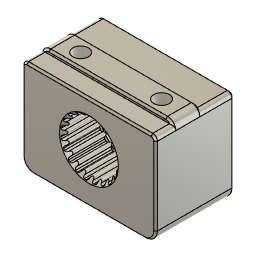
nozzle_probe (Autodesk Fusion 360 design; units mm, degrees)
Autodesk Fusion 360 part; units mm, degrees
sketch "Sketch1" plane through (0, 0, 0) normal (0, 0, 1) x (1, 0, 0)
  line L0 (14.5, -10.2) -> (-14.5, -10.2)
  line L1 (-14.5, -10.2) -> (-14.5, 10.2)
  line L2 (-14.5, 10.2) -> (14.5, 10.2)
  line L3 (14.5, 10.2) -> (14.5, -10.2)
  line L4 (14.5, -10.2) -> (-14.5, 10.2) construction
  line L5 (-14.5, -10.2) -> (14.5, 10.2) construction
  circle A0 centre (0, 0.6) radius 6.26
  dimension "d115" = 29
  dimension "d116" = 20.4
  dimension "d117" = 12.52
  dimension "d177" = 10.8
  constraint horizontal L0
  constraint perpendicular L0 L1
  constraint parallel L0 L2
  constraint parallel L1 L3
  constraint coincident L4 origin
  constraint coincident L5 origin
  constraint vertical origin A0.centre
  measures "d115" distance of L1.end L2.end
  measures "d116" distance of L0.start L2.end
  measures "d117" diameter of A0
  measures "d177" distance of L0 A0.centre
extrude "Extrude1" add sketch "Sketch1" along normal blind 17 contours L0 L1 L2 L3 | A0
sketch "Sketch6" plane through (0, 0, 17) normal (0, 0, 1) x (1, 0, 0)
  line L0 (14.5, 10.2) -> (-14.5, 10.2)
  line L1 (-14.5, 10.2) -> (-14.5, -10.2)
  line L2 (-14.5, -10.2) -> (14.5, -10.2)
  line L3 (14.5, -10.2) -> (14.5, 10.2)
  circle A0 centre (0, 0.6) radius 6.26
extrude "Extrude6" cut sketch "Sketch6" against normal blind 8 contours A0
sketch "Sketch7" plane through (0, 0, 17) normal (0, 0, 1) x (1, 0, 0)
  circle A0 centre (0, 0.6) radius 6.26
  line L0 (14.5, 10.2) -> (-14.5, 10.2)
  line L1 (-14.5, 10.2) -> (-14.5, -10.2)
  line L2 (-14.5, -10.2) -> (14.5, -10.2)
  line L3 (14.5, -10.2) -> (14.5, 10.2)
  circle A1 centre (0, 0.6) radius 6.26
  circle A2 centre (0, 0.6) radius 5.2
  dimension "d179" = 10.4
  constraint coincident A0.centre A1.centre
  measures "d179" diameter of A2
extrude "Extrude8" cut sketch "Sketch7" against normal blind 9 contours A2
sketch "Sketch2" plane through (0, 0, 17) normal (0, 0, 1) x (1, 0, 0)
  line L0 (14.5, 10.2) -> (-14.5, 10.2)
  line L1 (-14.5, 10.2) -> (-14.5, -10.2)
  line L2 (-14.5, -10.2) -> (14.5, -10.2)
  line L3 (14.5, -10.2) -> (14.5, 10.2)
  line L4 (0.4, 6.47) -> (0.4, 6.8472)
  line L5 (-0.4, 6.8472) -> (-0.4, 6.47)
  arc A0 (-0.4, 6.47) -> (0.4, 6.47) centre (0, 6.47) ccw
  circle A1 centre (0, 0.6) radius 6.26
  circle A2 centre (0, 0.6) radius 6.26
  dimension "d121" = 0.8
  dimension "d172" = 5.87
  constraint vertical L4
  constraint vertical L5
  constraint tangent L4 A0
  constraint tangent L5 A0
  constraint vertical A0.centre A1.centre
  constraint coincident L4.end A2
  constraint coincident L5.start A2
  measures "d121" diameter of A0
  measures "d172" distance of A0.centre A1.centre
extrude "Extrude2" add sketch "Sketch2" against normal blind 8 contours L4 L5 A0 A1 A2 picked at (-0.0445, 6.5995)
fillet "Fillet1" radius 0.35 2 edges at (-0.4, 6.8472, 13) (0.4, 6.8472, 13)
chamfer "Chamfer1" distance 0.4 angle 45 1 edges at (-4.8481, 2.4804, 9)
pattern_circular "C-Pattern1" count 20 over 360 about axis through (0, 0.6, 17) along (0, 0, -1) of 3 faces at (-0.5335, 6.7373, 14.3333) (-0.0042, 6.07, 14.2901) (0.5475, 6.7477, 14.3333)
sketch "Sketch3" plane through (0, 0, 0) normal (1, 0, 0) x (0, 0, -1)
  line L0 (-17, 7) -> (-15, 5)
  line L1 (-15, 5) -> (-17, 5)
  line L2 (-17, 5) -> (-17, 7)
  line L3 (-17, -10.2, -14.5) -> (-17, -10.2, 14.5)
  line L4 (-17, 10.2) -> (-17, 0.6)
  line L5 (-17, 0.6) -> (-17, 7)
  line L6 (-17, 6.3024) -> (-17, 5.7827)
  line L7 (-17, 6.751) -> (-17, 6.3024)
  line L8 (-17, 6.751) -> (-17, 6.8094)
  line L9 (-17, 6.8122) -> (-17, 6.4659)
  line L10 (-17, 6.4659) -> (-17, 6.8122)
  line L11 (-17, 6.751) -> (-17, 6.8094)
  line L12 (-17, 6.2936) -> (-17, 6.0552)
  line L13 (-17, 6.751) -> (-17, 6.3024)
  line L14 (-17, 6.0904) -> (-17, 5.5807)
  line L15 (-17, 5.5807) -> (-17, 4.9489)
  line L16 (-17, 5.2518) -> (-17, 5.1105)
  line L17 (-17, 4.8925) -> (-17, 5.1566)
  line L18 (-17, 4.8925) -> (-17, 4.3715)
  line L19 (-17, 4.3715) -> (-17, 3.6503)
  line L20 (-17, 3.789) -> (-17, 3.6071)
  line L21 (-17, 3.2743) -> (-17, 3.6071)
  line L22 (-17, 3.2743) -> (-17, 2.7931)
  line L23 (-17, 2.7931) -> (-17, 2.0139)
  line L24 (-17, 2.0483) -> (-17, 1.7633)
  line L25 (-17, 1.3944) -> (-17, 1.7633)
  line L26 (-17, 0.2) -> (-17, -0.1944)
  line L27 (-17, 1) -> (-17, 0.2)
  line L28 (-17, 1.3944) -> (-17, 1)
  line L29 (-17, -0.5633) -> (-17, -0.8483)
  line L30 (-17, -0.8139) -> (-17, -1.5931)
  line L31 (-17, -1.5931) -> (-17, -2.0743)
  line L32 (-17, -2.4071) -> (-17, -2.0743)
  line L33 (-17, -2.4071) -> (-17, -2.589)
  line L34 (-17, -2.4503) -> (-17, -3.1715)
  line L35 (-17, -3.1715) -> (-17, -3.6925)
  line L36 (-17, -3.9566) -> (-17, -3.6925)
  line L37 (-17, -3.9105) -> (-17, -4.0518)
  line L38 (-17, -3.7489) -> (-17, -4.3807)
  line L39 (-17, -4.3807) -> (-17, -4.8904)
  line L40 (-17, -5.06) -> (-17, -4.8904)
  line L41 (-17, -4.8552) -> (-17, -5.0936)
  line L42 (-17, -4.5827) -> (-17, -5.1024)
  line L43 (-17, -5.1024) -> (-17, -5.551)
  line L44 (-17, -5.6094) -> (-17, -5.551)
  line L45 (-17, -5.2659) -> (-17, -5.6122)
  line L46 (-17, -4.87) -> (-17, -5.2659)
  line L47 (-17, -5.2659) -> (-17, -5.6122)
  line L48 (-17, -5.6094) -> (-17, -5.551)
  line L49 (-17, -5.1024) -> (-17, -5.551)
  line L50 (-17, -4.5827) -> (-17, -5.1024)
  line L51 (-17, -4.8552) -> (-17, -5.0936)
  line L52 (-17, -5.06) -> (-17, -4.8904)
  line L53 (-17, -4.3807) -> (-17, -4.8904)
  line L54 (-17, -3.7489) -> (-17, -4.3807)
  line L55 (-17, -3.9105) -> (-17, -4.0518)
  line L56 (-17, -3.9566) -> (-17, -3.6925)
  line L57 (-17, -3.1715) -> (-17, -3.6925)
  line L58 (-17, -2.4503) -> (-17, -3.1715)
  line L59 (-17, -2.4071) -> (-17, -2.589)
  line L60 (-17, -2.4071) -> (-17, -2.0743)
  line L61 (-17, -1.5931) -> (-17, -2.0743)
  line L62 (-17, -0.8139) -> (-17, -1.5931)
  line L63 (-17, -0.5633) -> (-17, -0.8483)
  line L64 (-17, -0.5633) -> (-17, -0.1944)
  line L65 (-17, 1.3944) -> (-17, 1)
  line L66 (-17, 1) -> (-17, 0.2)
  line L67 (-17, 0.2) -> (-17, -0.1944)
  line L68 (-17, 2.0483) -> (-17, 1.7633)
  line L69 (-17, 2.7931) -> (-17, 2.0139)
  line L70 (-17, 3.2743) -> (-17, 2.7931)
  line L71 (-17, 3.2743) -> (-17, 3.6071)
  line L72 (-17, 3.789) -> (-17, 3.6071)
  line L73 (-17, 4.3715) -> (-17, 3.6503)
  line L74 (-17, 4.8925) -> (-17, 4.3715)
  line L75 (-17, 4.8925) -> (-17, 5.1566)
  line L76 (-17, 5.2518) -> (-17, 5.1105)
  line L77 (-17, 5.5807) -> (-17, 4.9489)
  line L78 (-17, 6.0904) -> (-17, 5.5807)
  line L79 (-17, 6.0904) -> (-17, 6.26)
  line L80 (-17, 6.2936) -> (-17, 6.0552)
  line L81 (-17, 6.0904) -> (-17, 6.26)
  line L82 (-17, -0.5633) -> (-17, -0.1944)
  line L83 (-17, 1.3944) -> (-17, 1.7633)
  point P0 (-17, 10.2)
  point P1 (-17, -10.2)
  dimension "d129" = 2
  dimension "d163" = 9.6
  dimension "d164" = 6.4
  constraint perpendicular L1 L2
  constraint equal L1 L2
  constraint vertical L2
  constraint coincident P0 L4.start
  constraint vertical L4
  constraint vertical L5
  constraint coincident L2 L0.start
  constraint coincident L0.start L2.end
  measures "d129" distance of L0.start L1.end
  measures "d163" distance of P0 L4.end
  measures "d164" distance of L4.end L0.start
revolve "Revolve1" cut sketch "Sketch3" angle 360 about axis through (0, 0.6, 17) along (0, 0, 1)
hole "Hole1" at (-8.8, -10.2, 10) direction (0, 1, 0) diameter 3.4 end through all counterbore diameter 6 counterbore depth 5
pattern_linear "R-Pattern1" count 2 spacing 17.6 along (1, 0, 0) of "Hole1"
sketch "Sketch4" plane through (0, -10.2, 0) normal (0, -1, 0) x (1, 0, 0)
  circle A0 centre (-8.8, 10) radius 3
  line L0 (14.5, 17) -> (-14.5, 17)
  line L1 (-14.5, 17) -> (-14.5, 0)
  line L2 (-14.5, 0) -> (14.5, 0)
  line L3 (14.5, 0) -> (14.5, 17)
  line L4 (-2.3342, 4.8) -> (1.0842, 10)
  line L5 (1.0842, 10) -> (2.3342, 10)
  line L6 (2.3342, 10) -> (-1.0842, 4.8)
  line L7 (-1.0842, 4.8) -> (-2.3342, 4.8)
  line L8 (0.0342, 10) -> (-1.2158, 10)
  line L9 (-1.2158, 10) -> (-2.925, 7.4)
  line L10 (-2.925, 7.4) -> (-1.675, 7.4)
  line L11 (-1.675, 7.4) -> (0.0342, 10)
  line L12 (1.675, 7.4) -> (2.925, 7.4)
  line L13 (-0.0342, 4.8) -> (1.675, 7.4)
  line L14 (2.925, 7.4) -> (1.2158, 4.8)
  line L15 (1.2158, 4.8) -> (-0.0342, 4.8)
  line L16 (1.0842, 10) -> (-1.0842, 4.8) construction
  line L17 (-2.3342, 4.8) -> (2.3342, 10) construction
  circle A1 centre (8.8, 10) radius 3
  point P0 (0, 7.4)
  dimension "d146" = 5.2
  dimension "d147" = 1.25
  dimension "d148" = 1.05
  dimension "d149" = 2.6
  dimension "d150" = 1.05
  dimension "d151" = 7.4
  dimension "d152" = 14.5
  dimension "d209" = 56.68
  constraint horizontal L5
  constraint horizontal L7
  constraint parallel L4 L6
  constraint parallel L5 L8
  constraint parallel L4 L9
  constraint parallel L5 L10
  constraint parallel L4 L11
  constraint equal L5 L8
  constraint horizontal L12
  constraint parallel L6 L13
  constraint parallel L13 L14
  constraint horizontal L15
  constraint collinear L7 L15
  constraint collinear L10 L12
  constraint equal L10 L15
  constraint midpoint L17 P0
  constraint collinear L5 L8
  measures "d146" distance of L5 L7
  measures "d147" distance of L4.end L5.end
  measures "d148" horizontal distance of L4.end L8.start
  measures "d149" distance of L8 L10
  measures "d150" distance of L6.end L13.start
  measures "d151" distance of L2 P0
  measures "d152" distance of L1 P0
  measures "d209" angle of L4 L7
extrude "Extrude3" cut sketch "Sketch4" against normal blind 1.6 contours L4 L5 L6 L7 | L8 L9 L10 L11 | L12 L13 L14 L15
sketch "Sketch5" plane through (0, 0, 0) normal (0, 0, -1) x (-1, 0, 0)
  line L0 (3.1, -7.8) -> (-3.1, -7.8)
  line L1 (-3.1, -7.8) -> (-3.1, 5.4)
  line L2 (3.1, 5.4) -> (3.1, -7.8)
  line L3 (14.5, -6.4) -> (3.1, -6.4)
  line L4 (3.1, -6.4) -> (3.1, 4)
  line L5 (3.1, 4) -> (14.5, 4)
  line L6 (14.5, 4) -> (14.5, -6.4)
  line L7 (-3.1, 5.4) -> (3.1, 5.4)
  line L8 (14.5, 10.2) -> (-14.5, 10.2)
  line L9 (-14.5, 10.2) -> (-14.5, -10.2)
  line L10 (-14.5, -10.2) -> (14.5, -10.2)
  line L11 (14.5, -10.2) -> (14.5, 10.2)
  line L12 (-3.1, -4.5) -> (3.1, -4.5)
  dimension "d156" = 6.2
  dimension "d157" = 13.2
  dimension "d158" = 11.4
  dimension "d159" = 10.4
  dimension "d160" = 1.4
  dimension "d175" = 9.9
  constraint horizontal L3
  constraint horizontal L5
  constraint vertical L6
  constraint coincident L2 L4.end
  constraint vertical L2
  constraint vertical L4
  constraint vertical L1
  constraint horizontal L7
  constraint coincident L1 L12.start
  constraint coincident L4 L12.end
  constraint horizontal L12
  measures "d156" distance of L0.start L0.end
  measures "d157" distance of L0.end L1.end
  measures "d158" distance of L3.start L3.end
  measures "d159" distance of L3.start L5.end
  measures "d160" distance of L0 L3
  measures "d175" distance of L7 L12
extrude "Extrude4" cut sketch "Sketch5" against normal blind 8.2 contours L0 L1 L2 L4 L12 | L1 L2 L4 L7 L12
extrude "Extrude5" cut sketch "Sketch5" against normal blind 6 contours L2 L3 L4 L5 L6 L11
extrude "Extrude7" cut sketch "Sketch5" against normal blind 9 contours L1 L2 L4 L7 L12
sketch "Sketch8" plane through (-14.5, -0.131, 0.0085) normal (-1, 0, 0) x (0, 0, 1)
  line L0 (-0.0085, 4.131) -> (5.9915, 4.131)
  line L1 (5.9915, 4.131) -> (5.9915, -6.269)
  line L2 (5.9915, -6.269) -> (-0.0085, -6.269)
  line L3 (-0.0085, -6.269) -> (-0.0085, -10.069)
  line L4 (-0.0085, -10.069) -> (16.9915, -10.069)
  line L5 (16.9915, -10.069) -> (16.9915, 10.331)
  line L6 (16.9915, 10.331) -> (-0.0085, 10.331)
  line L7 (-0.0085, 10.331) -> (-0.0085, 4.131)
  line L8 (5.9915, 4.131) -> (5.9915, -6.269)
  line L9 (5.9915, -1.069) -> (12.5209, -1.069)
  line L10 (5.9915, -2.844) -> (8.7915, -2.844)
  line L11 (8.7915, -2.844) -> (8.7915, 0.706)
  line L12 (8.7915, 0.706) -> (5.9915, 0.706)
  line L13 (5.9915, 0.706) -> (5.9915, -2.844)
  line L14 (5.9915, -2.844) -> (8.7915, 0.706) construction
  line L15 (8.7915, -2.844) -> (5.9915, 0.706) construction
  point P0 (7.3915, -1.069)
  dimension "d183" = 3.55
  dimension "d184" = 2.8
  constraint midpoint L1 L9.start
  constraint perpendicular L1 L9
  constraint horizontal L10
  constraint perpendicular L10 L11
  constraint parallel L10 L12
  constraint parallel L11 L13
  constraint coincident L14 P0
  constraint coincident L15 P0
  constraint coincident L9 P0
  constraint coincident L1 L10.start
  measures "d183" distance of L10.end L11.end
  measures "d184" distance of L10.start L10.end
extrude "Extrude9" cut sketch "Sketch8" against normal blind 3.4 contours L1 L8 L9 L11 L12 L13 | L1 L8 L9 L10 L11 L13
fillet "Fillet2" radius 1 2 edges at (-12.8, 0.575, 8.8) (-12.8, -2.975, 8.8)
hole "Hole2" at (3.1, 2.05, 3) direction (1, 0, 0) diameter 1.6 depth 5.6 tip angle 180
pattern_linear "R-Pattern2" count 2 spacing 6.5 along (0, -1, 0) of "Hole2"
sketch "Sketch9" plane through (0, 10.2, 0) normal (0, 1, 0) x (-1, 0, 0)
  circle A0 centre (-8.8, 10) radius 1.7
  circle A1 centre (8.8, 10) radius 1.7
  line L0 (-14.5, 0) -> (14.5, 0)
  line L1 (14.5, 0) -> (14.5, 17)
  line L2 (14.5, 17) -> (-14.5, 17)
  line L3 (-14.5, 17) -> (-14.5, 0)
  line L4 (-14.5, 13) -> (14.5, 13)
  line L5 (14.5, 13) -> (14.5, 7)
  line L6 (14.5, 7) -> (-14.5, 7)
  line L7 (-14.5, 7) -> (-14.5, 13)
  dimension "d198" = 7
  dimension "d199" = 6
  constraint horizontal L4
  constraint vertical L5
  constraint horizontal L6
  constraint vertical L7
  constraint coincident L1 L5.end
  constraint coincident L3 L4.start
  measures "d198" distance of L0 L6
  measures "d199" distance of L4.end L5.end
extrude "Extrude10" add sketch "Sketch9" along normal blind 0.8 contours L1 L3 L4 L5 L6 L7
fillet "Fillet3" radius 2.5 2 edges at (-14.5, -10.2, 8.5) (14.5, -10.2, 8.5)
fillet "Fillet3" radius 1 4 edges at (14.5, 10.2, 15) (14.5, 10.2, 3.5) (-14.5, 10.2, 15) (-14.5, 10.2, 3.5)
fillet "Fillet3" radius 1.8 2 edges at (-14.5, 11, 10) (14.5, 11, 10)
chamfer "Chamfer2" distance 0.4 angle 45 30 edges at (0, 11, 13) (-13.9728, 10.4728, 13) (13.9728, 10.4728, 13) (0, 11, 7) (13.9728, 10.4728, 7) (-13.9728, 10.4728, 7) (0, 10.2, 17) (-14.2071, 9.9071, 17) (-14.5, 0.75, 17) (-13.7678, -9.4678, 17) (0, -10.2, 17) (13.7678, -9.4678, 17) (14.5, 0.75, 17) (14.2071, 9.9071, 17) (0, 10.2, 0) (14.2071, 9.9071, 0) (14.5, 0.75, 0) (13.7678, -9.4678, 0) (0, -10.2, 0) (-13.7678, -9.4678, 0) (-14.5, -7.05, 0) (-14.5, 6.6, 0) (-14.2071, 9.9071, 0) (-3.1, 4.7, 0) (-8.8, 4, 0) (0, 5.4, 0) (3.1, -1.2, 0) (0, -7.8, 0) (-3.1, -7.1, 0) (-8.8, -6.4, 0)
sketch "Sketch10" plane through (0, 0, 6) normal (0, 0, -1) x (-1, 0, 0)
  line L0 (14.5, -2.975) -> (11.1, -2.975)
  line L1 (11.1, -2.975) -> (11.1, 0.575)
  line L2 (11.1, 0.575) -> (14.5, 0.575)
  line L3 (14.5, 0.575) -> (14.5, 4)
  line L4 (14.5, 4) -> (3.1, 4)
  line L5 (3.1, 4) -> (3.1, -6.4)
  line L6 (3.1, -6.4) -> (14.5, -6.4)
  line L7 (14.5, -6.4) -> (14.5, -2.975)
  line L8 (14.5, -6.4) -> (3.1, -6.4)
  line L9 (3.1, 4) -> (14.5, 4)
  line L10 (7.3, -6.4) -> (5.7, -6.4)
  line L11 (5.7, -6.4) -> (5.7, 4)
  line L12 (5.7, 4) -> (7.3, 4)
  line L13 (7.3, 4) -> (7.3, -6.4)
  dimension "d210" = 1.6
  dimension "d211" = 7.2
  constraint horizontal L10
  constraint vertical L11
  constraint horizontal L12
  constraint coincident L4 L11.end
  constraint coincident L6 L10.start
  measures "d210" distance of L10.start L10.end
  measures "d211" distance of L7 L13
extrude "Extrude11" add sketch "Sketch10" along normal blind 1 contours L4 L6 L8 L9 L10 L11 L12 L13
equation "d117 = ( 6.26 * 2 ) * 1 mm"
equation "d149 = d146 / 2"
equation "d150 = d148"
equation "d151 = 4.8 mm + 2.6 mm"
equation "d152 = ( 29 / 2 ) * 1 mm"
equation "d164 = ( 12.8 / 2 ) * 1 mm"
equation "d209 = 56.68 °"
